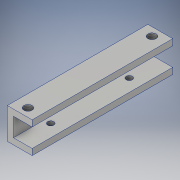
# Autodesk Inventor part: sensor3_lock
Saved by Autodesk Inventor 2018 (Build 220112000, 112)
## iProperties
Created: 2021-04-23
Part Number: sensor3_lock
Material: Aluminum 6061
Document SubType Name: Modeling
Designer: Ramana Bharathi
Mass: 17.8583 g
Surface Area: 51.4741 cm^2
Volume: 6.61419 cm^3
Density: 2.7 g/cm^3
Appearance: Aluminum - Flat
Author: Ramana Bharathi
Autodesk Inventor part; units mm, degrees
ref_plane "YZ Plane" through (0, 0, 0) normal (1, 0, 0) x (0, 1, 0)
ref_plane "XZ Plane" through (0, 0, 0) normal (0, 1, 0) x (-1, 0, 0)
ref_plane "XY Plane" through (0, 0, 0) normal (0, 0, 1) x (1, 0, 0)
sketch "Sketch1" plane through (0, 0, 0) normal (0, 1, 0) x (-1, 0, 0)
  line L0 (0, 0) -> (-12, 0)
  line L1 (-12, 0) -> (-12, -68)
  line L2 (-12, -68) -> (0, -68)
  line L3 (0, -68) -> (0, 0)
  dimension "d0" = 12
  dimension "d1" = 68
  constraints: 8 end point, 2 parallel, 1 horizontal, 1 perpendicular
  measures "d0" distance of L2.end L1.end
  measures "d1" distance of L1.end L0.end
extrude "Extrusion1" add sketch "Sketch1" along normal blind 15
sketch "Sketch4" plane through (12, 0, 0) normal (1, 0, 0) x (0, 0, -1)
  line L0 (0, 0) -> (0, 15) projected
  line L1 (0, 3) -> (68, 3)
  line L2 (68, 3) -> (68, 12)
  line L3 (68, 12) -> (0, 12)
  line L4 (0, 12) -> (0, 3)
  line L5 (0, 0) -> (68, 0) projected
  dimension "d30" = 68
  dimension "d31" = 9
  dimension "d32" = 3
  constraints: 8 end point, 2 parallel, 1 horizontal, 1 perpendicular, 1 point on line
  measures "d30" distance of L3.end L2.end
  measures "d31" distance of L2.end L1.end
  measures "d32" distance between parallel lines of L1 L5
extrude "Extrusion2" cut sketch "Sketch4" against normal blind 9
sketch "Sketch2" plane through (0, 15, 0) normal (0, 1, 0) x (1, 0, 0)
  circle A0 centre (6, 64) radius 2
  circle A1 centre (6, 4) radius 2
  line L0 (0, 68) -> (0, 0) projected
  line L1 (12, 68) -> (0, 68) projected
  line L2 (0, 0) -> (12, 0) projected
  dimension "d4" = 4
  dimension "d5" = 4
  dimension "d6" = 6
  dimension "d7" = 6
  dimension "d8" = 4
  dimension "d9" = 4
  constraints: 2 centre point
  measures "d4" diameter of A0
  measures "d5" diameter of A1
  measures "d6" distance from line of L0 A0.centre
  measures "d7" distance from line of L0 A1.centre
  measures "d8" distance from line of L1 A0.centre
  measures "d9" distance from line of L2 A1.centre
hole "Hole1" at (6, 15, -4) at (6, 15, -64) direction (0, -1, 0) diameter 4 depth 3 tip angle 118
sketch "Sketch3" plane through (0, 0, 0) normal (0, -1, 0) x (1, 0, 0)
  circle A0 centre (6, -15) radius 1.5
  circle A1 centre (6, -53) radius 1.5
  line L0 (0, -68) -> (0, 0) projected
  line L1 (0, 0) -> (12, 0) projected
  line L2 (12, -68) -> (0, -68) projected
  dimension "d17" = 3
  dimension "d18" = 3
  dimension "d19" = 6
  dimension "d20" = 6
  dimension "d21" = 15
  dimension "d22" = 15
  constraints: 2 centre point
  measures "d17" diameter of A0
  measures "d18" diameter of A1
  measures "d19" distance from line of L0 A0.centre
  measures "d20" distance from line of L0 A1.centre
  measures "d21" distance from line of L1 A0.centre
  measures "d22" distance from line of L2 A1.centre
hole "Hole2" at (6, 0, -53) at (6, 0, -15) direction (0, 1, 0) diameter 3 depth 3 tip angle 118
thread "Thread1" size "M4x0.7" class "6H" standard "ANSI Metric M Profile" full length
thread "Thread2" size "M4x0.7" class "6H" standard "ANSI Metric M Profile" full length
thread "Thread3" size "M3x0.5" class "6H" standard "ANSI Metric M Profile" full length
thread "Thread4" size "M3x0.5" class "6H" standard "ANSI Metric M Profile" full length
body "Solid1"
